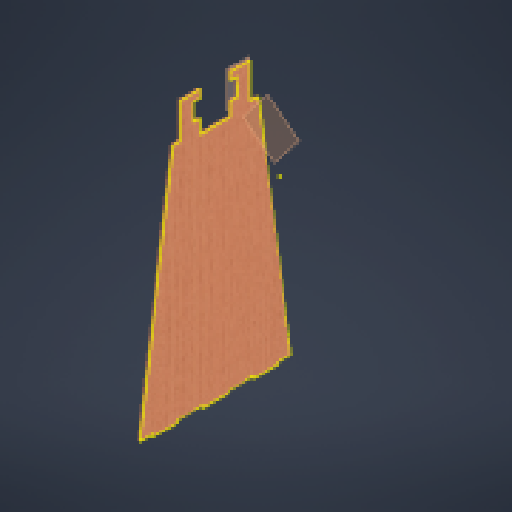
# Autodesk Inventor part: Stand 2
Saved by Autodesk Inventor 2025.2 (Build 292293000, 293)
## iProperties
Created: 2024-11-19
Part Number: Stand 2
Material: Wood (Oak)
Document SubType Name: Modeling
Designer: JL
Density: 0.76 g/cm^3
Appearance: White Oak - Natural Medium Gloss
Author: JL
Autodesk Inventor part; units mm, degrees
ref_plane "YZ Plane" through (0, 0, 0) normal (1, 0, 0) x (0, 1, 0)
ref_plane "XZ Plane" through (0, 0, 0) normal (0, 1, 0) x (-1, 0, 0)
ref_plane "XY Plane" through (0, 0, 0) normal (0, 0, 1) x (1, 0, 0)
ref_plane "Work Plane1" through (92.6217, 101.5189, 36.552) normal (1, 0, 0) x (0, 1, 0)
ref_plane "Work Plane2" through (89.5017, 946.6624, 79.752) normal (0, 0, 1) x (0.6133, 0.7899, 0)
sketch "Sketch1" plane through (92.6217, 101.5189, 36.552) normal (1, 0, 0) x (0, 1, 0)
  line L0 (31.35, 24.7) -> (31.35, 16.2) projected
  line L1 (31.35, 16.2) -> (9.35, 16.2) projected
  line L2 (9.35, 16.2) -> (9.35, 24.7) projected
  line L3 (0, 24.7) -> (9.35, 24.7) projected
  line L4 (0, 0) -> (0, 24.7) construction
  line L5 (40.7, 0) -> (0, 0) projected
  line L6 (40.7, 0) -> (40.7, 24.7) projected
  line L7 (31.35, 24.7) -> (40.7, 24.7) projected
  line L8 (9.35, 61.7) -> (9.35, 70.2) projected
  line L9 (9.35, 70.2) -> (31.35, 70.2) projected
  line L10 (31.35, 70.2) -> (31.35, 61.7) projected
  line L11 (31.35, 61.7) -> (40.7, 61.7) projected
  line L12 (40.7, 61.7) -> (40.7, 86.4) projected
  line L13 (40.7, 86.4) -> (0, 86.4) projected
  line L14 (0, 86.4) -> (0, 61.7) construction
  line L15 (0, 61.7) -> (9.35, 61.7) projected
  line L16 (-4.1716, 58.2) -> (44.8716, 58.2) projected
  line L17 (-4.1716, 28.2) -> (44.8716, 28.2) projected
  line L18 (-300, 136.4) -> (-300, 120.8667) projected
  line L19 (0, 61.7) -> (-4.1716, 61.7)
  line L20 (-4.1716, 61.7) -> (-7.6716, 61.7)
  line L21 (-7.6716, 61.7) -> (-7.6716, 43.2)
  line L22 (-4.1716, 58.2) -> (-4.1716, 61.7) construction
  line L23 (-372.5743, 43.2) -> (114.4459, 43.2) construction
  line L24 (0, 24.7) -> (-4.1716, 24.7)
  line L25 (-4.1716, 24.7) -> (-7.6716, 24.7)
  line L26 (-7.6716, 24.7) -> (-7.6716, 43.2)
  line L27 (0, 86.4) -> (-3, 86.4)
  line L28 (-3, 86.4) -> (-3, 96.4)
  line L29 (-3, 96.4) -> (-300, 136.4)
  line L30 (0, 0) -> (-3, 0)
  line L31 (-3, 0) -> (-3, -10)
  line L32 (-300, 120.8667) -> (-303, 120.8667) projected
  line L33 (-303, 120.8667) -> (-303, 89.8) projected
  line L34 (-303, 89.8) -> (-300, 89.8) projected
  line L35 (-300, 89.8) -> (-300, 58.7333) projected
  line L36 (-300, 58.7333) -> (-303, 58.7333) projected
  line L37 (-303, 58.7333) -> (-303, 27.6667) projected
  line L38 (-303, 27.6667) -> (-300, 27.6667) projected
  line L39 (-300, 27.6667) -> (-300, -3.4) projected
  line L40 (-300, -3.4) -> (-303, -3.4) projected
  line L41 (-303, -3.4) -> (-303, -34.4667) projected
  line L42 (-303, -34.4667) -> (-300, -34.4667) projected
  line L43 (-300, -34.4667) -> (-300, -50) projected
  line L44 (-300, -50) -> (-3, -10)
  point P0 (-101.5189, -36.552)
  dimension "d2" = 10
  dimension "d4" = 3
  constraints: 26 end point, 4 symmetric about line, 2 horizontal, 2 perpendicular, 2 point on line, 2 vertical
  measures "d2" distance of L27.end L28.end
  measures "d4" distance of L13.end L27.end
extrude "Extrusion1" add sketch "Sketch1" along normal blind 3
sketch "Sketch2" plane through (95.6217, 101.5189, 36.552) normal (1, 0, 0) x (0, 0, -1)
  line L0 (-24.7, 40.7) -> (-24.7, 31.35) projected
  line L1 (-24.7, 31.35) -> (-16.2, 31.35) projected
  line L2 (-16.2, 31.35) -> (-16.2, 9.35) projected
  line L3 (-16.2, 9.35) -> (-24.7, 9.35) projected
  line L4 (-24.7, 9.35) -> (-24.7, -7.6716) projected
  line L5 (-24.7, -7.6716) -> (-61.7, -7.6716) projected
  line L6 (-61.7, -7.6716) -> (-61.7, 9.35) projected
  line L7 (-61.7, 9.35) -> (-70.2, 9.35) projected
  line L8 (-70.2, 9.35) -> (-70.2, 31.35) projected
  line L9 (-70.2, 31.35) -> (-61.7, 31.35) projected
  line L10 (-61.7, 31.35) -> (-61.7, 40.7) projected
  line L11 (-61.7, 40.7) -> (-86.4, 40.7) projected
  line L12 (-86.4, 40.7) -> (-86.4, -3) projected
  line L13 (-86.4, -3) -> (-96.4, -3) projected
  line L14 (-96.4, -3) -> (-136.4, -300) projected
  line L15 (-136.4, -300) -> (-120.8667, -300) projected
  line L16 (-120.8667, -300) -> (-120.8667, -303) projected
  line L17 (-120.8667, -303) -> (-89.8, -303) projected
  line L18 (-89.8, -303) -> (-89.8, -300) projected
  line L19 (-89.8, -300) -> (-58.7333, -300) projected
  line L20 (-58.7333, -300) -> (-58.7333, -303) projected
  line L21 (-58.7333, -303) -> (-27.6667, -303) projected
  line L22 (-27.6667, -303) -> (-27.6667, -300) projected
  line L23 (-27.6667, -300) -> (3.4, -300) projected
  line L24 (3.4, -300) -> (3.4, -303) projected
  line L25 (3.4, -303) -> (34.4667, -303) projected
  line L26 (34.4667, -303) -> (34.4667, -300) projected
  line L27 (34.4667, -300) -> (50, -300) projected
  line L28 (50, -300) -> (10, -3) projected
  line L29 (10, -3) -> (0, -3) projected
  line L30 (0, -3) -> (0, 40.7) projected
  line L31 (0, 40.7) -> (-24.7, 40.7) projected
  point P0 (36.552, -101.5189)
body "Solid1"
